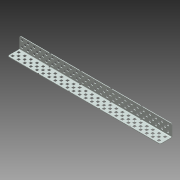
# Autodesk Inventor part: 275-1033
Saved by Autodesk Inventor 2013 (Build 170138000, 138)
## iProperties
Company: Autodesk Inc.
Category: Structure
Created: 2005-08-01
Part Number: 275-1033
Document SubType Name: Sheet Metal
Designer: Autodesk Inc.
Density: 7.85 g/cm^3
Sheet Metal Rule: Default
Catalog Web Link: http://www.vexrobotics.com/catalogsearch/result/?q=275-1033
Vendor: Innovation First, Inc.
Material: Steel
Mass: 122.685 g
Surface Area: 290.459 cm^2
Volume: 15.6287 cm^3
Author: Autodesk Inc.
Title: VEX Robotics Kit of Parts
Autodesk Inventor part; units mm, degrees
ref_plane "YZ Plane" through (0, 0, 0) normal (1, 0, 0) x (0, 1, 0)
ref_plane "XZ Plane" through (0, 0, 0) normal (0, 1, 0) x (-1, 0, 0)
ref_plane "XY Plane" through (0, 0, 0) normal (0, 0, 1) x (1, 0, 0)
sketch "Sketch1" plane through (0, 0, 0) normal (0, 0, 1) x (1, 0, 0)
  line L0 (-158.75, 22.86) -> (158.75, 22.86)
  line L1 (-155.956, 19.939) -> (-151.384, 19.939)
  line L2 (-151.384, 19.939) -> (-151.384, 15.367)
  line L3 (-151.384, 15.367) -> (-155.956, 15.367)
  line L4 (-155.956, 15.367) -> (-155.956, 19.939)
  line L5 (-155.956, 7.239) -> (-151.384, 7.239)
  line L6 (-151.384, 7.239) -> (-151.384, 2.667)
  line L7 (-151.384, 2.667) -> (-155.956, 2.667)
  line L8 (-155.956, 2.667) -> (-155.956, 7.239)
  line L9 (-143.256, 19.939) -> (-138.684, 19.939)
  line L10 (-138.684, 19.939) -> (-138.684, 15.367)
  line L11 (-138.684, 15.367) -> (-143.256, 15.367)
  line L12 (-143.256, 15.367) -> (-143.256, 19.939)
  line L13 (-143.256, 7.239) -> (-138.684, 7.239)
  line L14 (-138.684, 7.239) -> (-138.684, 2.667)
  line L15 (-138.684, 2.667) -> (-143.256, 2.667)
  line L16 (-143.256, 2.667) -> (-143.256, 7.239)
  line L17 (-149.606, 13.589) -> (-145.034, 13.589)
  line L18 (-145.034, 13.589) -> (-145.034, 9.017)
  line L19 (-145.034, 9.017) -> (-149.606, 9.017)
  line L20 (-149.606, 9.017) -> (-149.606, 13.589)
  line L21 (-130.556, 19.939) -> (-125.984, 19.939)
  line L22 (-125.984, 19.939) -> (-125.984, 15.367)
  line L23 (-125.984, 15.367) -> (-130.556, 15.367)
  line L24 (-130.556, 15.367) -> (-130.556, 19.939)
  line L25 (-130.556, 7.239) -> (-125.984, 7.239)
  line L26 (-125.984, 7.239) -> (-125.984, 2.667)
  line L27 (-125.984, 2.667) -> (-130.556, 2.667)
  line L28 (-130.556, 2.667) -> (-130.556, 7.239)
  line L29 (-136.906, 9.017) -> (-136.906, 13.589)
  line L30 (-136.906, 13.589) -> (-132.334, 13.589)
  line L31 (-132.334, 9.017) -> (-136.906, 9.017)
  line L32 (-132.334, 13.589) -> (-132.334, 9.017)
  line L33 (-117.856, 19.939) -> (-113.284, 19.939)
  line L34 (-113.284, 19.939) -> (-113.284, 15.367)
  line L35 (-113.284, 15.367) -> (-117.856, 15.367)
  line L36 (-117.856, 15.367) -> (-117.856, 19.939)
  line L37 (-117.856, 7.239) -> (-113.284, 7.239)
  line L38 (-113.284, 7.239) -> (-113.284, 2.667)
  line L39 (-113.284, 2.667) -> (-117.856, 2.667)
  line L40 (-117.856, 2.667) -> (-117.856, 7.239)
  line L41 (-124.206, 9.017) -> (-124.206, 13.589)
  line L42 (-124.206, 13.589) -> (-119.634, 13.589)
  line L43 (-119.634, 9.017) -> (-124.206, 9.017)
  line L44 (-119.634, 13.589) -> (-119.634, 9.017)
  line L45 (-105.156, 19.939) -> (-100.584, 19.939)
  line L46 (-100.584, 19.939) -> (-100.584, 15.367)
  line L47 (-100.584, 15.367) -> (-105.156, 15.367)
  line L48 (-105.156, 15.367) -> (-105.156, 19.939)
  line L49 (-105.156, 7.239) -> (-100.584, 7.239)
  line L50 (-100.584, 7.239) -> (-100.584, 2.667)
  line L51 (-100.584, 2.667) -> (-105.156, 2.667)
  line L52 (-105.156, 2.667) -> (-105.156, 7.239)
  line L53 (-111.506, 9.017) -> (-111.506, 13.589)
  line L54 (-111.506, 13.589) -> (-106.934, 13.589)
  line L55 (-106.934, 9.017) -> (-111.506, 9.017)
  line L56 (-106.934, 13.589) -> (-106.934, 9.017)
  line L57 (-92.456, 19.939) -> (-87.884, 19.939)
  line L58 (-87.884, 19.939) -> (-87.884, 15.367)
  line L59 (-87.884, 15.367) -> (-92.456, 15.367)
  line L60 (-92.456, 15.367) -> (-92.456, 19.939)
  line L61 (-92.456, 7.239) -> (-87.884, 7.239)
  line L62 (-87.884, 7.239) -> (-87.884, 2.667)
  line L63 (-87.884, 2.667) -> (-92.456, 2.667)
  line L64 (-92.456, 2.667) -> (-92.456, 7.239)
  line L65 (-98.806, 9.017) -> (-98.806, 13.589)
  line L66 (-98.806, 13.589) -> (-94.234, 13.589)
  line L67 (-94.234, 9.017) -> (-98.806, 9.017)
  line L68 (-94.234, 13.589) -> (-94.234, 9.017)
  line L69 (-79.756, 19.939) -> (-75.184, 19.939)
  line L70 (-75.184, 19.939) -> (-75.184, 15.367)
  line L71 (-75.184, 15.367) -> (-79.756, 15.367)
  line L72 (-79.756, 15.367) -> (-79.756, 19.939)
  line L73 (-79.756, 7.239) -> (-75.184, 7.239)
  line L74 (-75.184, 7.239) -> (-75.184, 2.667)
  line L75 (-75.184, 2.667) -> (-79.756, 2.667)
  line L76 (-79.756, 2.667) -> (-79.756, 7.239)
  line L77 (-86.106, 9.017) -> (-86.106, 13.589)
  line L78 (-86.106, 13.589) -> (-81.534, 13.589)
  line L79 (-81.534, 9.017) -> (-86.106, 9.017)
  line L80 (-81.534, 13.589) -> (-81.534, 9.017)
  line L81 (-67.056, 19.939) -> (-62.484, 19.939)
  line L82 (-62.484, 19.939) -> (-62.484, 15.367)
  line L83 (-62.484, 15.367) -> (-67.056, 15.367)
  line L84 (-67.056, 15.367) -> (-67.056, 19.939)
  line L85 (-67.056, 7.239) -> (-62.484, 7.239)
  line L86 (-62.484, 7.239) -> (-62.484, 2.667)
  line L87 (-62.484, 2.667) -> (-67.056, 2.667)
  line L88 (-67.056, 2.667) -> (-67.056, 7.239)
  line L89 (-73.406, 9.017) -> (-73.406, 13.589)
  line L90 (-73.406, 13.589) -> (-68.834, 13.589)
  line L91 (-68.834, 9.017) -> (-73.406, 9.017)
  line L92 (-68.834, 13.589) -> (-68.834, 9.017)
  line L93 (-54.356, 19.939) -> (-49.784, 19.939)
  line L94 (-49.784, 19.939) -> (-49.784, 15.367)
  line L95 (-49.784, 15.367) -> (-54.356, 15.367)
  line L96 (-54.356, 15.367) -> (-54.356, 19.939)
  line L97 (-54.356, 7.239) -> (-49.784, 7.239)
  line L98 (-49.784, 7.239) -> (-49.784, 2.667)
  line L99 (-49.784, 2.667) -> (-54.356, 2.667)
  line L100 (-54.356, 2.667) -> (-54.356, 7.239)
  line L101 (-60.706, 9.017) -> (-60.706, 13.589)
  line L102 (-60.706, 13.589) -> (-56.134, 13.589)
  line L103 (-56.134, 9.017) -> (-60.706, 9.017)
  line L104 (-56.134, 13.589) -> (-56.134, 9.017)
  line L105 (-41.656, 19.939) -> (-37.084, 19.939)
  line L106 (-37.084, 19.939) -> (-37.084, 15.367)
  line L107 (-37.084, 15.367) -> (-41.656, 15.367)
  line L108 (-41.656, 15.367) -> (-41.656, 19.939)
  line L109 (-41.656, 7.239) -> (-37.084, 7.239)
  line L110 (-37.084, 7.239) -> (-37.084, 2.667)
  line L111 (-37.084, 2.667) -> (-41.656, 2.667)
  line L112 (-41.656, 2.667) -> (-41.656, 7.239)
  line L113 (-48.006, 9.017) -> (-48.006, 13.589)
  line L114 (-48.006, 13.589) -> (-43.434, 13.589)
  line L115 (-43.434, 9.017) -> (-48.006, 9.017)
  line L116 (-43.434, 13.589) -> (-43.434, 9.017)
  line L117 (-28.956, 19.939) -> (-24.384, 19.939)
  line L118 (-24.384, 19.939) -> (-24.384, 15.367)
  line L119 (-24.384, 15.367) -> (-28.956, 15.367)
  line L120 (-28.956, 15.367) -> (-28.956, 19.939)
  line L121 (-28.956, 7.239) -> (-24.384, 7.239)
  line L122 (-24.384, 7.239) -> (-24.384, 2.667)
  line L123 (-24.384, 2.667) -> (-28.956, 2.667)
  line L124 (-28.956, 2.667) -> (-28.956, 7.239)
  line L125 (-35.306, 9.017) -> (-35.306, 13.589)
  line L126 (-35.306, 13.589) -> (-30.734, 13.589)
  line L127 (-30.734, 9.017) -> (-35.306, 9.017)
  line L128 (-30.734, 13.589) -> (-30.734, 9.017)
  line L129 (-16.256, 19.939) -> (-11.684, 19.939)
  line L130 (-11.684, 19.939) -> (-11.684, 15.367)
  line L131 (-11.684, 15.367) -> (-16.256, 15.367)
  line L132 (-16.256, 15.367) -> (-16.256, 19.939)
  line L133 (-16.256, 7.239) -> (-11.684, 7.239)
  line L134 (-11.684, 7.239) -> (-11.684, 2.667)
  line L135 (-11.684, 2.667) -> (-16.256, 2.667)
  line L136 (-16.256, 2.667) -> (-16.256, 7.239)
  line L137 (-22.606, 9.017) -> (-22.606, 13.589)
  line L138 (-22.606, 13.589) -> (-18.034, 13.589)
  line L139 (-18.034, 9.017) -> (-22.606, 9.017)
  line L140 (-18.034, 13.589) -> (-18.034, 9.017)
  line L141 (-3.556, 19.939) -> (1.016, 19.939)
  line L142 (1.016, 19.939) -> (1.016, 15.367)
  line L143 (1.016, 15.367) -> (-3.556, 15.367)
  line L144 (-3.556, 15.367) -> (-3.556, 19.939)
  line L145 (-3.556, 7.239) -> (1.016, 7.239)
  line L146 (1.016, 7.239) -> (1.016, 2.667)
  line L147 (1.016, 2.667) -> (-3.556, 2.667)
  line L148 (-3.556, 2.667) -> (-3.556, 7.239)
  line L149 (-9.906, 9.017) -> (-9.906, 13.589)
  line L150 (-9.906, 13.589) -> (-5.334, 13.589)
  line L151 (-5.334, 9.017) -> (-9.906, 9.017)
  line L152 (-5.334, 13.589) -> (-5.334, 9.017)
  line L153 (9.144, 19.939) -> (13.716, 19.939)
  line L154 (13.716, 19.939) -> (13.716, 15.367)
  line L155 (13.716, 15.367) -> (9.144, 15.367)
  line L156 (9.144, 15.367) -> (9.144, 19.939)
  line L157 (9.144, 7.239) -> (13.716, 7.239)
  line L158 (13.716, 7.239) -> (13.716, 2.667)
  line L159 (13.716, 2.667) -> (9.144, 2.667)
  line L160 (9.144, 2.667) -> (9.144, 7.239)
  line L161 (2.794, 9.017) -> (2.794, 13.589)
  line L162 (2.794, 13.589) -> (7.366, 13.589)
  line L163 (7.366, 9.017) -> (2.794, 9.017)
  line L164 (7.366, 13.589) -> (7.366, 9.017)
  line L165 (21.844, 19.939) -> (26.416, 19.939)
  line L166 (26.416, 19.939) -> (26.416, 15.367)
  line L167 (26.416, 15.367) -> (21.844, 15.367)
  line L168 (21.844, 15.367) -> (21.844, 19.939)
  line L169 (21.844, 7.239) -> (26.416, 7.239)
  line L170 (26.416, 7.239) -> (26.416, 2.667)
  line L171 (26.416, 2.667) -> (21.844, 2.667)
  line L172 (21.844, 2.667) -> (21.844, 7.239)
  line L173 (15.494, 9.017) -> (15.494, 13.589)
  line L174 (15.494, 13.589) -> (20.066, 13.589)
  line L175 (20.066, 9.017) -> (15.494, 9.017)
  line L176 (20.066, 13.589) -> (20.066, 9.017)
  line L177 (34.544, 19.939) -> (39.116, 19.939)
  line L178 (39.116, 19.939) -> (39.116, 15.367)
  line L179 (39.116, 15.367) -> (34.544, 15.367)
  line L180 (34.544, 15.367) -> (34.544, 19.939)
  line L181 (34.544, 7.239) -> (39.116, 7.239)
  line L182 (39.116, 7.239) -> (39.116, 2.667)
  line L183 (39.116, 2.667) -> (34.544, 2.667)
  line L184 (34.544, 2.667) -> (34.544, 7.239)
  line L185 (28.194, 9.017) -> (28.194, 13.589)
  line L186 (28.194, 13.589) -> (32.766, 13.589)
  line L187 (32.766, 9.017) -> (28.194, 9.017)
  line L188 (32.766, 13.589) -> (32.766, 9.017)
  line L189 (158.75, 22.86) -> (158.75, 0)
  line L190 (158.75, 0) -> (-158.75, 0)
  line L191 (-158.75, 0) -> (-158.75, 22.86)
  line L192 (47.244, 19.939) -> (51.816, 19.939)
  line L193 (51.816, 19.939) -> (51.816, 15.367)
  line L194 (51.816, 15.367) -> (47.244, 15.367)
  line L195 (47.244, 15.367) -> (47.244, 19.939)
  line L196 (47.244, 7.239) -> (51.816, 7.239)
  line L197 (51.816, 7.239) -> (51.816, 2.667)
  line L198 (51.816, 2.667) -> (47.244, 2.667)
  line L199 (47.244, 2.667) -> (47.244, 7.239)
  line L200 (40.894, 9.017) -> (40.894, 13.589)
  line L201 (40.894, 13.589) -> (45.466, 13.589)
  line L202 (45.466, 9.017) -> (40.894, 9.017)
  line L203 (45.466, 13.589) -> (45.466, 9.017)
  line L204 (59.944, 19.939) -> (64.516, 19.939)
  line L205 (64.516, 19.939) -> (64.516, 15.367)
  line L206 (64.516, 15.367) -> (59.944, 15.367)
  line L207 (59.944, 15.367) -> (59.944, 19.939)
  line L208 (59.944, 7.239) -> (64.516, 7.239)
  line L209 (64.516, 7.239) -> (64.516, 2.667)
  line L210 (64.516, 2.667) -> (59.944, 2.667)
  line L211 (59.944, 2.667) -> (59.944, 7.239)
  line L212 (53.594, 9.017) -> (53.594, 13.589)
  line L213 (53.594, 13.589) -> (58.166, 13.589)
  line L214 (58.166, 9.017) -> (53.594, 9.017)
  line L215 (58.166, 13.589) -> (58.166, 9.017)
  line L216 (72.644, 19.939) -> (77.216, 19.939)
  line L217 (77.216, 19.939) -> (77.216, 15.367)
  line L218 (77.216, 15.367) -> (72.644, 15.367)
  line L219 (72.644, 15.367) -> (72.644, 19.939)
  line L220 (72.644, 7.239) -> (77.216, 7.239)
  line L221 (77.216, 7.239) -> (77.216, 2.667)
  line L222 (77.216, 2.667) -> (72.644, 2.667)
  line L223 (72.644, 2.667) -> (72.644, 7.239)
  line L224 (66.294, 9.017) -> (66.294, 13.589)
  line L225 (66.294, 13.589) -> (70.866, 13.589)
  line L226 (70.866, 9.017) -> (66.294, 9.017)
  line L227 (70.866, 13.589) -> (70.866, 9.017)
  line L228 (85.344, 19.939) -> (89.916, 19.939)
  line L229 (89.916, 19.939) -> (89.916, 15.367)
  line L230 (89.916, 15.367) -> (85.344, 15.367)
  line L231 (85.344, 15.367) -> (85.344, 19.939)
  line L232 (85.344, 7.239) -> (89.916, 7.239)
  line L233 (89.916, 7.239) -> (89.916, 2.667)
  line L234 (89.916, 2.667) -> (85.344, 2.667)
  line L235 (85.344, 2.667) -> (85.344, 7.239)
  line L236 (78.994, 9.017) -> (78.994, 13.589)
  line L237 (78.994, 13.589) -> (83.566, 13.589)
  line L238 (83.566, 9.017) -> (78.994, 9.017)
  line L239 (83.566, 13.589) -> (83.566, 9.017)
  line L240 (98.044, 19.939) -> (102.616, 19.939)
  line L241 (102.616, 19.939) -> (102.616, 15.367)
  line L242 (102.616, 15.367) -> (98.044, 15.367)
  line L243 (98.044, 15.367) -> (98.044, 19.939)
  line L244 (98.044, 7.239) -> (102.616, 7.239)
  line L245 (102.616, 7.239) -> (102.616, 2.667)
  line L246 (102.616, 2.667) -> (98.044, 2.667)
  line L247 (98.044, 2.667) -> (98.044, 7.239)
  line L248 (91.694, 9.017) -> (91.694, 13.589)
  line L249 (91.694, 13.589) -> (96.266, 13.589)
  line L250 (96.266, 9.017) -> (91.694, 9.017)
  line L251 (96.266, 13.589) -> (96.266, 9.017)
  line L252 (110.744, 19.939) -> (115.316, 19.939)
  line L253 (115.316, 19.939) -> (115.316, 15.367)
  line L254 (115.316, 15.367) -> (110.744, 15.367)
  line L255 (110.744, 15.367) -> (110.744, 19.939)
  line L256 (110.744, 7.239) -> (115.316, 7.239)
  line L257 (115.316, 7.239) -> (115.316, 2.667)
  line L258 (115.316, 2.667) -> (110.744, 2.667)
  line L259 (110.744, 2.667) -> (110.744, 7.239)
  line L260 (104.394, 9.017) -> (104.394, 13.589)
  line L261 (104.394, 13.589) -> (108.966, 13.589)
  line L262 (108.966, 9.017) -> (104.394, 9.017)
  line L263 (108.966, 13.589) -> (108.966, 9.017)
  line L264 (123.444, 19.939) -> (128.016, 19.939)
  line L265 (128.016, 19.939) -> (128.016, 15.367)
  line L266 (128.016, 15.367) -> (123.444, 15.367)
  line L267 (123.444, 15.367) -> (123.444, 19.939)
  line L268 (123.444, 7.239) -> (128.016, 7.239)
  line L269 (128.016, 7.239) -> (128.016, 2.667)
  line L270 (128.016, 2.667) -> (123.444, 2.667)
  line L271 (123.444, 2.667) -> (123.444, 7.239)
  line L272 (117.094, 9.017) -> (117.094, 13.589)
  line L273 (117.094, 13.589) -> (121.666, 13.589)
  line L274 (121.666, 9.017) -> (117.094, 9.017)
  line L275 (121.666, 13.589) -> (121.666, 9.017)
  line L276 (136.144, 19.939) -> (140.716, 19.939)
  line L277 (140.716, 19.939) -> (140.716, 15.367)
  line L278 (140.716, 15.367) -> (136.144, 15.367)
  line L279 (136.144, 15.367) -> (136.144, 19.939)
  line L280 (136.144, 7.239) -> (140.716, 7.239)
  line L281 (140.716, 7.239) -> (140.716, 2.667)
  line L282 (140.716, 2.667) -> (136.144, 2.667)
  line L283 (136.144, 2.667) -> (136.144, 7.239)
  line L284 (129.794, 9.017) -> (129.794, 13.589)
  line L285 (129.794, 13.589) -> (134.366, 13.589)
  line L286 (134.366, 9.017) -> (129.794, 9.017)
  line L287 (134.366, 13.589) -> (134.366, 9.017)
  line L288 (148.844, 19.939) -> (153.416, 19.939)
  line L289 (153.416, 19.939) -> (153.416, 15.367)
  line L290 (153.416, 15.367) -> (148.844, 15.367)
  line L291 (148.844, 15.367) -> (148.844, 19.939)
  line L292 (148.844, 7.239) -> (153.416, 7.239)
  line L293 (153.416, 7.239) -> (153.416, 2.667)
  line L294 (153.416, 2.667) -> (148.844, 2.667)
  line L295 (148.844, 2.667) -> (148.844, 7.239)
  line L296 (142.494, 9.017) -> (142.494, 13.589)
  line L297 (142.494, 13.589) -> (147.066, 13.589)
  line L298 (147.066, 9.017) -> (142.494, 9.017)
  line L299 (147.066, 13.589) -> (147.066, 9.017)
  point P0 (0, 0)
  point P1 (0, 0)
  dimension "d13" = 12.7
  dimension "d20" = 2.794
  dimension "d22" = 2.921
  dimension "d23" = 22.86
  dimension "d24" = 4.572
  dimension "d25" = 8.128
  dimension "d26" = 4.572
  dimension "d125" = 317.5
  dimension "d126" = 4.572
  dimension "d127" = 4.572
  dimension "d128" = 4.572
  dimension "d129" = 9.017
  dimension "d130" = 9.144
  dimension "d133" = 15.494
  dimension "d134" = 4.572
  measures "d20" distance between parallel lines of L191 L4
  measures "d22" distance between parallel lines of L0 L1
  measures "d23" distance between parallel lines of L190 L0
  measures "d24" distance of L3.end L1.start
  measures "d25" distance between parallel lines of L5 L3
  measures "d26" distance of L7.end L5.start
  measures "d125" distance of L189.end L190.end
  measures "d126" distance of L1.start L1.end
  measures "d127" distance of L20.end L17.end
  measures "d128" distance of L17.end L19.start
  measures "d129" distance between parallel lines of L190 L19
  measures "d130" distance between parallel lines of L191 L20
  measures "d133" distance between parallel lines of L191 L12
  measures "d134" distance of L9.start L9.end
extrude "Plate9" add sketch "Sketch1" along normal blind 1.27
sketch "Sketch14" plane through (158.75, -1.27, 2.54) normal (0, -1, 0) x (1, 0, 0)
  line L0 (-317.5, 0) -> (0, 0)
  line L1 (0, 0) -> (0, 22.86)
  line L2 (0, 22.86) -> (-317.5, 22.86)
  line L3 (-317.5, 22.86) -> (-317.5, 0)
  constraints: 6 end point, 1 horizontal, 1 perpendicular, 1 vertical
edge flange "Flange8" height 25.4 angle 90 thickness 1.27 bend radius 1.27 thickness toward (0, -1, 0) relief tear relief width 1.27 relief depth 0.635 edges at (0, 0, 1.27) wall of the first edge with corners at (-158.75, -1.27, 2.54) (158.75, -1.27, 2.54) (158.75, -1.27, 25.4) (-158.75, -1.27, 25.4)
bend "Bend8"
corner "Corner1"
sketch "Sketch15" plane through (-158.75, -1.27, 25.4) normal (0, 1, 0) x (1, 0, 0)
  line L0 (0, 0) -> (0, 22.86) projected
  line L1 (0, 0) -> (317.5, 0) projected
  line L2 (2.794, 2.921) -> (7.366, 2.921)
  line L3 (7.366, 2.921) -> (7.366, 7.493)
  line L4 (7.366, 7.493) -> (2.794, 7.493)
  line L5 (2.794, 7.493) -> (2.794, 2.921)
  line L6 (2.794, 15.621) -> (7.366, 15.621)
  line L7 (7.366, 15.621) -> (7.366, 20.193)
  line L8 (7.366, 20.193) -> (2.794, 20.193)
  line L9 (2.794, 20.193) -> (2.794, 15.621)
  line L10 (9.144, 9.017) -> (13.716, 9.017)
  line L11 (13.716, 9.017) -> (13.716, 13.589)
  line L12 (13.716, 13.589) -> (9.144, 13.589)
  line L13 (9.144, 13.589) -> (9.144, 9.017)
  line L14 (15.494, 15.621) -> (20.066, 15.621)
  line L15 (20.066, 15.621) -> (20.066, 20.193)
  line L16 (20.066, 20.193) -> (15.494, 20.193)
  line L17 (15.494, 20.193) -> (15.494, 15.621)
  line L18 (15.494, 7.493) -> (20.066, 7.493)
  line L19 (20.066, 7.493) -> (20.066, 2.921)
  line L20 (20.066, 2.921) -> (15.494, 2.921)
  line L21 (15.494, 2.921) -> (15.494, 7.493)
  line L22 (21.844, 9.017) -> (26.416, 9.017)
  line L23 (26.416, 9.017) -> (26.416, 13.589)
  line L24 (26.416, 13.589) -> (21.844, 13.589)
  line L25 (21.844, 13.589) -> (21.844, 9.017)
  line L26 (28.194, 15.621) -> (32.766, 15.621)
  line L27 (32.766, 15.621) -> (32.766, 20.193)
  line L28 (32.766, 20.193) -> (28.194, 20.193)
  line L29 (28.194, 20.193) -> (28.194, 15.621)
  line L30 (28.194, 7.493) -> (32.766, 7.493)
  line L31 (32.766, 7.493) -> (32.766, 2.921)
  line L32 (32.766, 2.921) -> (28.194, 2.921)
  line L33 (28.194, 2.921) -> (28.194, 7.493)
  line L34 (34.544, 9.017) -> (39.116, 9.017)
  line L35 (39.116, 9.017) -> (39.116, 13.589)
  line L36 (39.116, 13.589) -> (34.544, 13.589)
  line L37 (34.544, 13.589) -> (34.544, 9.017)
  line L38 (40.894, 15.621) -> (45.466, 15.621)
  line L39 (45.466, 15.621) -> (45.466, 20.193)
  line L40 (45.466, 20.193) -> (40.894, 20.193)
  line L41 (40.894, 20.193) -> (40.894, 15.621)
  line L42 (40.894, 7.493) -> (45.466, 7.493)
  line L43 (45.466, 7.493) -> (45.466, 2.921)
  line L44 (45.466, 2.921) -> (40.894, 2.921)
  line L45 (40.894, 2.921) -> (40.894, 7.493)
  line L46 (47.244, 9.017) -> (51.816, 9.017)
  line L47 (51.816, 9.017) -> (51.816, 13.589)
  line L48 (51.816, 13.589) -> (47.244, 13.589)
  line L49 (47.244, 13.589) -> (47.244, 9.017)
  line L50 (53.594, 15.621) -> (58.166, 15.621)
  line L51 (58.166, 15.621) -> (58.166, 20.193)
  line L52 (58.166, 20.193) -> (53.594, 20.193)
  line L53 (53.594, 20.193) -> (53.594, 15.621)
  line L54 (53.594, 7.493) -> (58.166, 7.493)
  line L55 (58.166, 7.493) -> (58.166, 2.921)
  line L56 (58.166, 2.921) -> (53.594, 2.921)
  line L57 (53.594, 2.921) -> (53.594, 7.493)
  line L58 (59.944, 9.017) -> (64.516, 9.017)
  line L59 (64.516, 9.017) -> (64.516, 13.589)
  line L60 (64.516, 13.589) -> (59.944, 13.589)
  line L61 (59.944, 13.589) -> (59.944, 9.017)
  line L62 (66.294, 15.621) -> (70.866, 15.621)
  line L63 (70.866, 15.621) -> (70.866, 20.193)
  line L64 (70.866, 20.193) -> (66.294, 20.193)
  line L65 (66.294, 20.193) -> (66.294, 15.621)
  line L66 (66.294, 7.493) -> (70.866, 7.493)
  line L67 (70.866, 7.493) -> (70.866, 2.921)
  line L68 (70.866, 2.921) -> (66.294, 2.921)
  line L69 (66.294, 2.921) -> (66.294, 7.493)
  line L70 (72.644, 9.017) -> (77.216, 9.017)
  line L71 (77.216, 9.017) -> (77.216, 13.589)
  line L72 (77.216, 13.589) -> (72.644, 13.589)
  line L73 (72.644, 13.589) -> (72.644, 9.017)
  line L74 (78.994, 15.621) -> (83.566, 15.621)
  line L75 (83.566, 15.621) -> (83.566, 20.193)
  line L76 (83.566, 20.193) -> (78.994, 20.193)
  line L77 (78.994, 20.193) -> (78.994, 15.621)
  line L78 (78.994, 7.493) -> (83.566, 7.493)
  line L79 (83.566, 7.493) -> (83.566, 2.921)
  line L80 (83.566, 2.921) -> (78.994, 2.921)
  line L81 (78.994, 2.921) -> (78.994, 7.493)
  line L82 (85.344, 9.017) -> (89.916, 9.017)
  line L83 (89.916, 9.017) -> (89.916, 13.589)
  line L84 (89.916, 13.589) -> (85.344, 13.589)
  line L85 (85.344, 13.589) -> (85.344, 9.017)
  line L86 (91.694, 15.621) -> (96.266, 15.621)
  line L87 (96.266, 15.621) -> (96.266, 20.193)
  line L88 (96.266, 20.193) -> (91.694, 20.193)
  line L89 (91.694, 20.193) -> (91.694, 15.621)
  line L90 (91.694, 7.493) -> (96.266, 7.493)
  line L91 (96.266, 7.493) -> (96.266, 2.921)
  line L92 (96.266, 2.921) -> (91.694, 2.921)
  line L93 (91.694, 2.921) -> (91.694, 7.493)
  line L94 (98.044, 9.017) -> (102.616, 9.017)
  line L95 (102.616, 9.017) -> (102.616, 13.589)
  line L96 (102.616, 13.589) -> (98.044, 13.589)
  line L97 (98.044, 13.589) -> (98.044, 9.017)
  line L98 (104.394, 15.621) -> (108.966, 15.621)
  line L99 (108.966, 15.621) -> (108.966, 20.193)
  line L100 (108.966, 20.193) -> (104.394, 20.193)
  line L101 (104.394, 20.193) -> (104.394, 15.621)
  line L102 (104.394, 7.493) -> (108.966, 7.493)
  line L103 (108.966, 7.493) -> (108.966, 2.921)
  line L104 (108.966, 2.921) -> (104.394, 2.921)
  line L105 (104.394, 2.921) -> (104.394, 7.493)
  line L106 (110.744, 9.017) -> (115.316, 9.017)
  line L107 (115.316, 9.017) -> (115.316, 13.589)
  line L108 (115.316, 13.589) -> (110.744, 13.589)
  line L109 (110.744, 13.589) -> (110.744, 9.017)
  line L110 (117.094, 15.621) -> (121.666, 15.621)
  line L111 (121.666, 15.621) -> (121.666, 20.193)
  line L112 (121.666, 20.193) -> (117.094, 20.193)
  line L113 (117.094, 20.193) -> (117.094, 15.621)
  line L114 (117.094, 7.493) -> (121.666, 7.493)
  line L115 (121.666, 7.493) -> (121.666, 2.921)
  line L116 (121.666, 2.921) -> (117.094, 2.921)
  line L117 (117.094, 2.921) -> (117.094, 7.493)
  line L118 (123.444, 9.017) -> (128.016, 9.017)
  line L119 (128.016, 9.017) -> (128.016, 13.589)
  line L120 (128.016, 13.589) -> (123.444, 13.589)
  line L121 (123.444, 13.589) -> (123.444, 9.017)
  line L122 (129.794, 15.621) -> (134.366, 15.621)
  line L123 (134.366, 15.621) -> (134.366, 20.193)
  line L124 (134.366, 20.193) -> (129.794, 20.193)
  line L125 (129.794, 20.193) -> (129.794, 15.621)
  line L126 (129.794, 7.493) -> (134.366, 7.493)
  line L127 (134.366, 7.493) -> (134.366, 2.921)
  line L128 (134.366, 2.921) -> (129.794, 2.921)
  line L129 (129.794, 2.921) -> (129.794, 7.493)
  line L130 (136.144, 9.017) -> (140.716, 9.017)
  line L131 (140.716, 9.017) -> (140.716, 13.589)
  line L132 (140.716, 13.589) -> (136.144, 13.589)
  line L133 (136.144, 13.589) -> (136.144, 9.017)
  line L134 (142.494, 15.621) -> (147.066, 15.621)
  line L135 (147.066, 15.621) -> (147.066, 20.193)
  line L136 (147.066, 20.193) -> (142.494, 20.193)
  line L137 (142.494, 20.193) -> (142.494, 15.621)
  line L138 (142.494, 7.493) -> (147.066, 7.493)
  line L139 (147.066, 7.493) -> (147.066, 2.921)
  line L140 (147.066, 2.921) -> (142.494, 2.921)
  line L141 (142.494, 2.921) -> (142.494, 7.493)
  line L142 (148.844, 9.017) -> (153.416, 9.017)
  line L143 (153.416, 9.017) -> (153.416, 13.589)
  line L144 (153.416, 13.589) -> (148.844, 13.589)
  line L145 (148.844, 13.589) -> (148.844, 9.017)
  line L146 (155.194, 15.621) -> (159.766, 15.621)
  line L147 (159.766, 15.621) -> (159.766, 20.193)
  line L148 (159.766, 20.193) -> (155.194, 20.193)
  line L149 (155.194, 20.193) -> (155.194, 15.621)
  line L150 (155.194, 7.493) -> (159.766, 7.493)
  line L151 (159.766, 7.493) -> (159.766, 2.921)
  line L152 (159.766, 2.921) -> (155.194, 2.921)
  line L153 (155.194, 2.921) -> (155.194, 7.493)
  line L154 (161.544, 9.017) -> (166.116, 9.017)
  line L155 (166.116, 9.017) -> (166.116, 13.589)
  line L156 (166.116, 13.589) -> (161.544, 13.589)
  line L157 (161.544, 13.589) -> (161.544, 9.017)
  line L158 (167.894, 15.621) -> (172.466, 15.621)
  line L159 (172.466, 15.621) -> (172.466, 20.193)
  line L160 (172.466, 20.193) -> (167.894, 20.193)
  line L161 (167.894, 20.193) -> (167.894, 15.621)
  line L162 (167.894, 7.493) -> (172.466, 7.493)
  line L163 (172.466, 7.493) -> (172.466, 2.921)
  line L164 (172.466, 2.921) -> (167.894, 2.921)
  line L165 (167.894, 2.921) -> (167.894, 7.493)
  line L166 (174.244, 9.017) -> (178.816, 9.017)
  line L167 (178.816, 9.017) -> (178.816, 13.589)
  line L168 (178.816, 13.589) -> (174.244, 13.589)
  line L169 (174.244, 13.589) -> (174.244, 9.017)
  line L170 (180.594, 15.621) -> (185.166, 15.621)
  line L171 (185.166, 15.621) -> (185.166, 20.193)
  line L172 (185.166, 20.193) -> (180.594, 20.193)
  line L173 (180.594, 20.193) -> (180.594, 15.621)
  line L174 (180.594, 7.493) -> (185.166, 7.493)
  line L175 (185.166, 7.493) -> (185.166, 2.921)
  line L176 (185.166, 2.921) -> (180.594, 2.921)
  line L177 (180.594, 2.921) -> (180.594, 7.493)
  line L178 (186.944, 9.017) -> (191.516, 9.017)
  line L179 (191.516, 9.017) -> (191.516, 13.589)
  line L180 (191.516, 13.589) -> (186.944, 13.589)
  line L181 (186.944, 13.589) -> (186.944, 9.017)
  line L182 (193.294, 15.621) -> (197.866, 15.621)
  line L183 (197.866, 15.621) -> (197.866, 20.193)
  line L184 (197.866, 20.193) -> (193.294, 20.193)
  line L185 (193.294, 20.193) -> (193.294, 15.621)
  line L186 (193.294, 7.493) -> (197.866, 7.493)
  line L187 (197.866, 7.493) -> (197.866, 2.921)
  line L188 (197.866, 2.921) -> (193.294, 2.921)
  line L189 (193.294, 2.921) -> (193.294, 7.493)
  line L190 (199.644, 9.017) -> (204.216, 9.017)
  line L191 (204.216, 9.017) -> (204.216, 13.589)
  line L192 (204.216, 13.589) -> (199.644, 13.589)
  line L193 (199.644, 13.589) -> (199.644, 9.017)
  line L194 (205.994, 15.621) -> (210.566, 15.621)
  line L195 (210.566, 15.621) -> (210.566, 20.193)
  line L196 (210.566, 20.193) -> (205.994, 20.193)
  line L197 (205.994, 20.193) -> (205.994, 15.621)
  line L198 (205.994, 7.493) -> (210.566, 7.493)
  line L199 (210.566, 7.493) -> (210.566, 2.921)
  line L200 (210.566, 2.921) -> (205.994, 2.921)
  line L201 (205.994, 2.921) -> (205.994, 7.493)
  line L202 (212.344, 9.017) -> (216.916, 9.017)
  line L203 (216.916, 9.017) -> (216.916, 13.589)
  line L204 (216.916, 13.589) -> (212.344, 13.589)
  line L205 (212.344, 13.589) -> (212.344, 9.017)
  line L206 (218.694, 15.621) -> (223.266, 15.621)
  line L207 (223.266, 15.621) -> (223.266, 20.193)
  line L208 (223.266, 20.193) -> (218.694, 20.193)
  line L209 (218.694, 20.193) -> (218.694, 15.621)
  line L210 (218.694, 7.493) -> (223.266, 7.493)
  line L211 (223.266, 7.493) -> (223.266, 2.921)
  line L212 (223.266, 2.921) -> (218.694, 2.921)
  line L213 (218.694, 2.921) -> (218.694, 7.493)
  line L214 (225.044, 9.017) -> (229.616, 9.017)
  line L215 (229.616, 9.017) -> (229.616, 13.589)
  line L216 (229.616, 13.589) -> (225.044, 13.589)
  line L217 (225.044, 13.589) -> (225.044, 9.017)
  line L218 (231.394, 15.621) -> (235.966, 15.621)
  line L219 (235.966, 15.621) -> (235.966, 20.193)
  line L220 (235.966, 20.193) -> (231.394, 20.193)
  line L221 (231.394, 20.193) -> (231.394, 15.621)
  line L222 (231.394, 7.493) -> (235.966, 7.493)
  line L223 (235.966, 7.493) -> (235.966, 2.921)
  line L224 (235.966, 2.921) -> (231.394, 2.921)
  line L225 (231.394, 2.921) -> (231.394, 7.493)
  line L226 (237.744, 9.017) -> (242.316, 9.017)
  line L227 (242.316, 9.017) -> (242.316, 13.589)
  line L228 (242.316, 13.589) -> (237.744, 13.589)
  line L229 (237.744, 13.589) -> (237.744, 9.017)
  line L230 (244.094, 15.621) -> (248.666, 15.621)
  line L231 (248.666, 15.621) -> (248.666, 20.193)
  line L232 (248.666, 20.193) -> (244.094, 20.193)
  line L233 (244.094, 20.193) -> (244.094, 15.621)
  line L234 (244.094, 7.493) -> (248.666, 7.493)
  line L235 (248.666, 7.493) -> (248.666, 2.921)
  line L236 (248.666, 2.921) -> (244.094, 2.921)
  line L237 (244.094, 2.921) -> (244.094, 7.493)
  line L238 (250.444, 9.017) -> (255.016, 9.017)
  line L239 (255.016, 9.017) -> (255.016, 13.589)
  line L240 (255.016, 13.589) -> (250.444, 13.589)
  line L241 (250.444, 13.589) -> (250.444, 9.017)
  line L242 (256.794, 15.621) -> (261.366, 15.621)
  line L243 (261.366, 15.621) -> (261.366, 20.193)
  line L244 (261.366, 20.193) -> (256.794, 20.193)
  line L245 (256.794, 20.193) -> (256.794, 15.621)
  line L246 (256.794, 7.493) -> (261.366, 7.493)
  line L247 (261.366, 7.493) -> (261.366, 2.921)
  line L248 (261.366, 2.921) -> (256.794, 2.921)
  line L249 (256.794, 2.921) -> (256.794, 7.493)
  line L250 (263.144, 9.017) -> (267.716, 9.017)
  line L251 (267.716, 9.017) -> (267.716, 13.589)
  line L252 (267.716, 13.589) -> (263.144, 13.589)
  line L253 (263.144, 13.589) -> (263.144, 9.017)
  line L254 (269.494, 15.621) -> (274.066, 15.621)
  line L255 (274.066, 15.621) -> (274.066, 20.193)
  line L256 (274.066, 20.193) -> (269.494, 20.193)
  line L257 (269.494, 20.193) -> (269.494, 15.621)
  line L258 (269.494, 7.493) -> (274.066, 7.493)
  line L259 (274.066, 7.493) -> (274.066, 2.921)
  line L260 (274.066, 2.921) -> (269.494, 2.921)
  line L261 (269.494, 2.921) -> (269.494, 7.493)
  line L262 (275.844, 9.017) -> (280.416, 9.017)
  line L263 (280.416, 9.017) -> (280.416, 13.589)
  line L264 (280.416, 13.589) -> (275.844, 13.589)
  line L265 (275.844, 13.589) -> (275.844, 9.017)
  line L266 (282.194, 15.621) -> (286.766, 15.621)
  line L267 (286.766, 15.621) -> (286.766, 20.193)
  line L268 (286.766, 20.193) -> (282.194, 20.193)
  line L269 (282.194, 20.193) -> (282.194, 15.621)
  line L270 (282.194, 7.493) -> (286.766, 7.493)
  line L271 (286.766, 7.493) -> (286.766, 2.921)
  line L272 (286.766, 2.921) -> (282.194, 2.921)
  line L273 (282.194, 2.921) -> (282.194, 7.493)
  line L274 (288.544, 9.017) -> (293.116, 9.017)
  line L275 (293.116, 9.017) -> (293.116, 13.589)
  line L276 (293.116, 13.589) -> (288.544, 13.589)
  line L277 (288.544, 13.589) -> (288.544, 9.017)
  line L278 (294.894, 15.621) -> (299.466, 15.621)
  line L279 (299.466, 15.621) -> (299.466, 20.193)
  line L280 (299.466, 20.193) -> (294.894, 20.193)
  line L281 (294.894, 20.193) -> (294.894, 15.621)
  line L282 (294.894, 7.493) -> (299.466, 7.493)
  line L283 (299.466, 7.493) -> (299.466, 2.921)
  line L284 (299.466, 2.921) -> (294.894, 2.921)
  line L285 (294.894, 2.921) -> (294.894, 7.493)
  line L286 (301.244, 9.017) -> (305.816, 9.017)
  line L287 (305.816, 9.017) -> (305.816, 13.589)
  line L288 (305.816, 13.589) -> (301.244, 13.589)
  line L289 (301.244, 13.589) -> (301.244, 9.017)
  line L290 (307.594, 15.621) -> (312.166, 15.621)
  line L291 (312.166, 15.621) -> (312.166, 20.193)
  line L292 (312.166, 20.193) -> (307.594, 20.193)
  line L293 (307.594, 20.193) -> (307.594, 15.621)
  line L294 (307.594, 7.493) -> (312.166, 7.493)
  line L295 (312.166, 7.493) -> (312.166, 2.921)
  line L296 (312.166, 2.921) -> (307.594, 2.921)
  line L297 (307.594, 2.921) -> (307.594, 7.493)
  point P0 (158.75, 25.4)
  dimension "d148" = 2.921
  dimension "d149" = 4.572
  dimension "d150" = 8.128
  dimension "d151" = 4.572
  dimension "d152" = 2.794
  dimension "d153" = 4.572
  dimension "d154" = 9.144
  dimension "d155" = 4.572
  dimension "d156" = 4.572
  dimension "d157" = 15.494
  dimension "d158" = 4.572
  dimension "d159" = 9.017
  dimension "d162" = 12.7
  constraints: 592 end point, 10 parallel, 8 collinear, 6 horizontal, 5 perpendicular, 552 other
  measures "d148" distance between parallel lines of L1 L2
  measures "d149" distance of L4.end L2.start
  measures "d150" distance between parallel lines of L6 L4
  measures "d151" distance of L8.end L6.start
  measures "d152" distance between parallel lines of L0 L5
  measures "d153" distance of L2.start L2.end
  measures "d154" distance between parallel lines of L0 L13
  measures "d155" distance of L10.start L10.end
  measures "d156" distance of L12.end L10.start
  measures "d157" distance between parallel lines of L0 L17
  measures "d158" distance of L15.end L16.end
  measures "d159" distance between parallel lines of L1 L10
  measures "d162" distance of L18.end L31.start
extrude "Cut4" cut sketch "Sketch15" against normal blind 1.27
sketch "Sketch16" plane through (0, 0, 1.27) normal (0, 0, 1) x (1, 0, 0)
  line L0 (-158.75, 22.86) -> (158.75, 22.86) projected
  line L1 (-158.75, 0) -> (-158.75, 22.86) projected
  line L2 (158.75, 0) -> (-158.75, 0) projected
  line L3 (-158.75, 20.955) -> (-156.845, 22.86)
  line L4 (-156.845, 22.86) -> (-160.655, 22.86)
  line L5 (-160.655, 22.86) -> (-158.75, 20.955)
  line L6 (-95.25, 20.955) -> (-93.345, 22.86)
  line L7 (-93.345, 22.86) -> (-97.155, 22.86)
  line L8 (-97.155, 22.86) -> (-95.25, 20.955)
  line L9 (-31.75, 20.955) -> (-29.845, 22.86)
  line L10 (-29.845, 22.86) -> (-33.655, 22.86)
  line L11 (-33.655, 22.86) -> (-31.75, 20.955)
  line L12 (31.75, 20.955) -> (33.655, 22.86)
  line L13 (33.655, 22.86) -> (29.845, 22.86)
  line L14 (29.845, 22.86) -> (31.75, 20.955)
  line L15 (95.25, 20.955) -> (97.155, 22.86)
  line L16 (97.155, 22.86) -> (93.345, 22.86)
  line L17 (93.345, 22.86) -> (95.25, 20.955)
  line L18 (158.75, 20.955) -> (160.655, 22.86)
  line L19 (160.655, 22.86) -> (156.845, 22.86)
  line L20 (156.845, 22.86) -> (158.75, 20.955)
  point P0 (0, 0)
  dimension "d169" = 1.905
  dimension "d172" = 63.5
  constraints: 36 end point, 2 perpendicular, 2 point on line, 1 horizontal, 1 parallel, 30 other
  measures "d169" horizontal distance of L3.start L3.end
  measures "d172" distance of L3.end L6.end
extrude "Cut5" cut sketch "Sketch16" against normal blind 1.27 contours L0 L3 L1 | L0 L6 L8 | L0 L9 L11 | L0 L12 L14 | L0 L15 L17 | L0 L19 L18 L20
sketch "Sketch17" plane through (-158.75, -1.27, 25.4) normal (0, 1, 0) x (1, 0, 0)
  line L0 (0, 0) -> (0, 22.86) projected
  line L1 (0, 0) -> (317.5, 0) construction
  line L2 (317.5, 0) -> (317.5, 22.86) projected
  line L3 (0, 1.905) -> (1.905, 0)
  line L4 (1.905, 0) -> (-1.905, 0)
  line L5 (-1.905, 0) -> (0, 1.905)
  line L6 (63.5, 1.905) -> (65.405, 0)
  line L7 (65.405, 0) -> (61.595, 0)
  line L8 (61.595, 0) -> (63.5, 1.905)
  line L9 (127, 1.905) -> (128.905, 0)
  line L10 (128.905, 0) -> (125.095, 0)
  line L11 (125.095, 0) -> (127, 1.905)
  line L12 (190.5, 1.905) -> (192.405, 0)
  line L13 (192.405, 0) -> (188.595, 0)
  line L14 (188.595, 0) -> (190.5, 1.905)
  line L15 (254, 1.905) -> (255.905, 0)
  line L16 (255.905, 0) -> (252.095, 0)
  line L17 (252.095, 0) -> (254, 1.905)
  line L18 (317.5, 1.905) -> (319.405, 0)
  line L19 (319.405, 0) -> (315.595, 0)
  line L20 (315.595, 0) -> (317.5, 1.905)
  point P0 (158.75, 25.4)
  dimension "d179" = 1.905
  dimension "d182" = 63.5
  constraints: 36 end point, 3 perpendicular, 2 point on line, 1 horizontal, 30 other
  measures "d179" horizontal distance of L4.end L3.start
  measures "d182" distance of L3.end L6.end
extrude "Cut6" cut sketch "Sketch17" against normal blind 1.27
sketch "Sketch18" plane through (-158.75, -1.27, 2.54) normal (0, 1, 0) x (1, 0, 0)
  line L0 (317.5, 0) -> (0, 0) projected
  line L1 (65.405, -22.86) -> (125.095, -22.86) projected
  line L2 (61.595, 1.1176) -> (63.5, -0.7874)
  line L3 (63.5, -0.7874) -> (65.405, 1.1176)
  line L4 (65.405, 1.1176) -> (63.5, 3.0226)
  line L5 (63.5, 3.0226) -> (61.595, 1.1176)
  line L6 (125.095, 1.1176) -> (127, -0.7874)
  line L7 (127, -0.7874) -> (128.905, 1.1176)
  line L8 (128.905, 1.1176) -> (127, 3.0226)
  line L9 (127, 3.0226) -> (125.095, 1.1176)
  line L10 (188.595, 1.1176) -> (190.5, -0.7874)
  line L11 (190.5, -0.7874) -> (192.405, 1.1176)
  line L12 (192.405, 1.1176) -> (190.5, 3.0226)
  line L13 (190.5, 3.0226) -> (188.595, 1.1176)
  line L14 (252.095, 1.1176) -> (254, -0.7874)
  line L15 (254, -0.7874) -> (255.905, 1.1176)
  line L16 (255.905, 1.1176) -> (254, 3.0226)
  line L17 (254, 3.0226) -> (252.095, 1.1176)
  point P0 (63.5, -20.955)
  point P1 (158.75, 2.54)
  dimension "d189" = 1.1176
  dimension "d190" = 1.905
  dimension "d193" = 63.5
  constraints: 32 end point, 2 parallel, 2 perpendicular, 1 horizontal, 1 horizontal alignment, 1 vertical alignment, 24 other
  measures "d189" distance from line of L0 L2.start
  measures "d190" horizontal distance of L4.end L2.start
  measures "d193" distance of L3.end L8.start
cut across bends "Cut7" sketch "Sketch18" k factor 0.44
sketch "Sketch19" plane through (0, 0, 1.27) normal (0, 0, 1) x (1, 0, 0)
  line L0 (-151.384, 19.939) -> (-151.384, 15.367) projected
  line L1 (-151.384, 15.367) -> (-155.956, 15.367) projected
  line L2 (-155.956, 15.367) -> (-155.956, 19.939) projected
  line L3 (-155.956, 19.939) -> (-151.384, 19.939) projected
  circle A0 centre (-153.67, 17.653) radius 2.286
  point P0 (0, 0)
  constraints: 4 tangent, 1 centre point
surface extrude "ExtrusionSrf1" sketch "Sketch19" against normal up to surface (1.27 mm away) shown no curves A0
pattern_linear "Rectangular Pattern1" count 25 spacing 12.7 along (1, 0, 0) count 2 spacing 12.7 along (0, -1, 0) of "ExtrusionSrf1"
sketch "Sketch20" plane through (0, 0, 1.27) normal (0, 0, 1) x (1, 0, 0)
  line L0 (-149.606, 9.017) -> (-149.606, 13.589) projected
  line L1 (-149.606, 13.589) -> (-145.034, 13.589) projected
  line L2 (-145.034, 13.589) -> (-145.034, 9.017) projected
  line L3 (-145.034, 9.017) -> (-149.606, 9.017) projected
  circle A0 centre (-147.32, 11.303) radius 2.286
  point P0 (0, 0)
  constraints: 4 tangent, 1 centre point
surface extrude "ExtrusionSrf51" sketch "Sketch20" against normal up to surface (1.27 mm away) shown no curves A0
pattern_linear "Rectangular Pattern2" count 24 spacing 12.7 along (1, 0, 0) of "ExtrusionSrf51"
sketch "Sketch21" plane through (97.155, -2.54, 25.4) normal (0, -1, 0) x (1, 0, 0)
  line L0 (51.689, -20.193) -> (51.689, -15.621) projected
  line L1 (51.689, -15.621) -> (56.261, -15.621) projected
  line L2 (56.261, -15.621) -> (56.261, -20.193) projected
  line L3 (56.261, -20.193) -> (51.689, -20.193) projected
  circle A0 centre (53.975, -17.907) radius 2.286
  point P0 (-97.155, -25.4)
  constraints: 4 tangent, 1 centre point
surface extrude "ExtrusionSrf75" sketch "Sketch21" against normal up to surface (1.27 mm away) shown no curves A0
pattern_linear "Rectangular Pattern3" count 25 spacing 12.7 along (-1, 0, 0) count 2 spacing 12.7 along (0, 0, 1) of "ExtrusionSrf75"
sketch "Sketch22" plane through (97.155, -2.54, 25.4) normal (0, -1, 0) x (1, 0, 0)
  line L0 (49.911, -9.017) -> (49.911, -13.589) projected
  line L1 (49.911, -13.589) -> (45.339, -13.589) projected
  line L2 (45.339, -13.589) -> (45.339, -9.017) projected
  line L3 (45.339, -9.017) -> (49.911, -9.017) projected
  circle A0 centre (47.625, -11.303) radius 2.286
  point P0 (-97.155, -25.4)
  constraints: 4 tangent, 1 centre point
surface extrude "ExtrusionSrf125" sketch "Sketch22" against normal up to surface (1.27 mm away) shown no curves A0
pattern_linear "Rectangular Pattern4" count 24 spacing 12.7 along (-1, 0, 0) of "ExtrusionSrf125"
equation "\"d167\" = Thickness"
equation "\"d177\" = Thickness"
equation "\"d187\" = Thickness"
equation "\"d138\" = BendReliefWidth"
equation "\"d139\" = BendReliefDepth"
equation "\"d140\" = MinimumRemnant"
equation "\"d141\" = BendRadius"
equation "\"d144\" = BendRadius"
equation "\"d145\" = CornerReliefSize"
equation "\"d146\" = GapSize"
equation "\"d147\" = JacobiRadiusSize"
equation "\"BendRadius\" = Thickness"
equation "\"BendReliefWidth\" = Thickness"
equation "\"BendReliefDepth\" = 0.5 * Thickness"
equation "\"CornerReliefSize\" = 4 * Thickness"
equation "\"MinimumRemnant\" = 2 * Thickness"
equation "\"TransitionRadius\" = BendRadius"
equation "\"d27\" = BendRadius"
equation "\"JacobiRadiusSize\" = BendRadius"
equation "\"GapSize\" = Thickness"
equation "\"d136\" = BendRadius"
equation "\"Thickness\" = 1.27"
body "Solid1"
body "Srf1"
body "Srf2"
body "Srf3"
body "Srf4"
body "Srf5"
body "Srf6"
body "Srf7"
body "Srf8"
body "Srf9"
body "Srf10"
body "Srf11"
body "Srf12"
body "Srf13"
body "Srf14"
body "Srf15"
body "Srf16"
body "Srf17"
body "Srf18"
body "Srf19"
body "Srf20"
body "Srf21"
body "Srf22"
body "Srf23"
body "Srf24"
body "Srf25"
body "Srf26"
body "Srf27"
body "Srf28"
body "Srf29"
body "Srf30"
body "Srf31"
body "Srf32"
body "Srf33"
body "Srf34"
body "Srf35"
body "Srf36"
body "Srf37"
body "Srf38"
body "Srf39"
body "Srf40"
body "Srf41"
body "Srf42"
body "Srf43"
body "Srf44"
body "Srf45"
body "Srf46"
body "Srf47"
body "Srf48"
body "Srf49"
body "Srf50"
body "Srf51"
body "Srf52"
body "Srf53"
body "Srf54"
body "Srf55"
body "Srf56"
body "Srf57"
body "Srf58"
body "Srf59"
body "Srf60"
body "Srf61"
body "Srf62"
body "Srf63"
body "Srf64"
body "Srf65"
body "Srf66"
body "Srf67"
body "Srf68"
body "Srf69"
body "Srf70"
body "Srf71"
body "Srf72"
body "Srf73"
body "Srf74"
body "Srf75"
body "Srf76"
body "Srf77"
body "Srf78"
body "Srf79"
body "Srf80"
body "Srf81"
body "Srf82"
body "Srf83"
body "Srf84"
body "Srf85"
body "Srf86"
body "Srf87"
body "Srf88"
body "Srf89"
body "Srf90"
body "Srf91"
body "Srf92"
body "Srf93"
body "Srf94"
body "Srf95"
body "Srf96"
body "Srf97"
body "Srf98"
body "Srf99"
body "Srf100"
body "Srf101"
body "Srf102"
body "Srf103"
body "Srf104"
body "Srf105"
body "Srf106"
body "Srf107"
body "Srf108"
body "Srf109"
body "Srf110"
body "Srf111"
body "Srf112"
body "Srf113"
body "Srf114"
body "Srf115"
body "Srf116"
body "Srf117"
body "Srf118"
body "Srf119"
body "Srf120"
body "Srf121"
body "Srf122"
body "Srf123"
body "Srf124"
body "Srf125"
body "Srf126"
body "Srf127"
body "Srf128"
body "Srf129"
body "Srf130"
body "Srf131"
body "Srf132"
body "Srf133"
body "Srf134"
body "Srf135"
body "Srf136"
body "Srf137"
body "Srf138"
body "Srf139"
body "Srf140"
body "Srf141"
body "Srf142"
body "Srf143"
body "Srf144"
body "Srf145"
body "Srf146"
body "Srf147"
body "Srf148"
